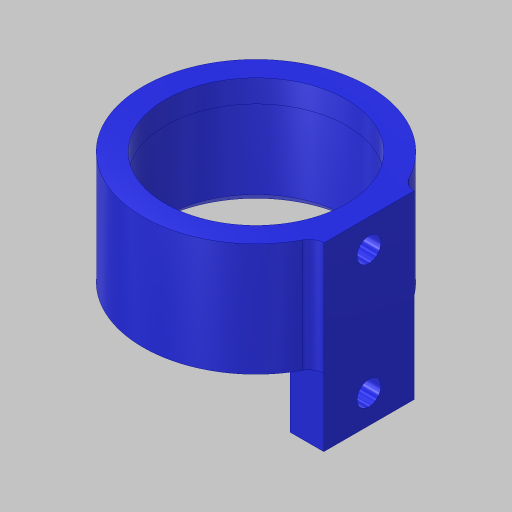
# Autodesk Inventor part: WL-008
Saved by Autodesk Inventor 2023.5 (Build 275446000, 446)
## iProperties
Created: 2025-02-22
Part Number: WL-008
Material: Aluminum 6061
Document SubType Name: Modeling
Designer: slick
Density: 2.7 g/cm^3
Appearance: Blue - Wall Paint - Glossy
Author: slick
Autodesk Inventor part; units mm, degrees
ref_plane "XZ Plane" through (0, 0, 0) normal (0, 1, 0) x (-1, 0, 0)
ref_plane "XY Plane" through (0, 0, 0) normal (0, 0, 1) x (1, 0, 0)
sketch "Sketch1" plane through (0, 0, 0) normal (0, 1, 0) x (-1, 0, 0)
  circle A0 centre (0, 0) radius 25.4
  circle A1 centre (0, 0) radius 31.75
  dimension "d0" = 50.8
  dimension "d1" = 63.5
  constraints: 2 centre point, 2 coincident
  measures "d0" diameter of A0
  measures "d1" diameter of A1
extrude "Extrusion1" add sketch "Sketch1" along normal blind 6.35
sketch "Sketch2" plane through (0, 0, 0) normal (0, -1, 0) x (1, 0, 0)
  circle A0 centre (0, 0) radius 25.654
  circle A1 centre (0, 0) radius 31.75 projected
  dimension "d4" = 51.308
  constraints: 1 centre point, 1 coincident
  measures "d4" diameter of A0
extrude "Extrusion2" add sketch "Sketch2" along normal blind 25.4
chamfer "Chamfer1" distance 3.175 angle 45 1 edges at (-25.654, -25.4, 0)
ref_plane "Work Plane1" through (31.75, 0, 0) normal (1, 0, 0) x (0, 1, 0)
sketch "Sketch5" plane through (31.75, 0, 0) normal (1, 0, 0) x (0, 1, 0)
  line L0 (-3.175, 31.75) -> (-34.925, 31.75) construction
  line L1 (-34.925, -31.75) -> (-3.175, -31.75) construction
  line L2 (-3.175, 31.75) -> (-34.925, -31.75) construction
  line L3 (-34.925, 31.75) -> (-3.175, -31.75) construction
  line L4 (0, 25.654) -> (0, -25.654) construction
  circle A0 centre (-19.05, 25.4) radius 3.35 construction
  circle A1 centre (-19.05, -25.4) radius 3.35 construction
  line L5 (-19.05, 25.4) -> (-19.05, -25.4) construction
  line L6 (-3.175, 31.75) -> (-3.175, -31.75) construction
  line L7 (-34.925, 31.75) -> (-34.925, -31.75) construction
  line L8 (-44.45, -12.7) -> (6.35, -12.7)
  line L9 (6.35, -12.7) -> (6.35, 12.7)
  line L10 (6.35, 12.7) -> (-44.45, 12.7)
  line L11 (-44.45, 12.7) -> (-44.45, -12.7)
  line L12 (-44.45, -12.7) -> (6.35, 12.7) construction
  line L13 (6.35, -12.7) -> (-44.45, 12.7) construction
  circle A2 centre (-1.5875, 0) radius 3.35
  circle A3 centre (-36.5125, 0) radius 3.35
  line L14 (-25.4, 31.75) -> (-25.4, -31.75) construction
  line L15 (6.35, -31.75) -> (6.35, 31.75) construction
  line L16 (6.35, -31.75) -> (6.35, 31.75) construction
  line L17 (6.35, 31.75) -> (-25.4, 31.75) construction
  line L18 (-25.4, 31.75) -> (6.35, 31.75) construction
  line L19 (-1.5875, 0) -> (-36.5125, 0) construction
  point P0 (0, 0)
  point P1 (6.35, 0)
  point P2 (-19.05, 0)
  point P3 (6.35, 0)
  point P4 (6.35, 0)
  point P5 (-9.525, 31.75)
  point P6 (-19.05, 0)
  point P7 (-44.45, 0)
  dimension "d27" = 63.5
  dimension "d28" = 50.8
  dimension "d29" = 6.7
  dimension "d35" = 25.4
  dimension "d36" = 34.925
  dimension "d37" = 50.8
  constraints: 30 end point, 10 midpoint, 4 centre point, 4 equal length, 4 horizontal alignment, 3 equal radius, 3 horizontal, 3 perpendicular, 1 coincident, 1 collinear, 1 vertical
  measures "d27" distance of L0.end L1.start
  measures "d28" distance of L5.start L5.end
  measures "d29" diameter of A0
  measures "d35" distance of L8.end L9.end
  measures "d36" distance of L19.start L19.end
  measures "d37" distance of point (-44.45, 0) point (6.35, 0)
extrude "Extrusion4" add sketch "Sketch5" against normal up to surface round surface about axis through (0, 0, 0) along (0, -1, 0) radius 25.654 far side no
extrude "Extrusion5" cut sketch "Sketch5" against normal blind 25.4 contours A2 | A3
fillet "Fillet1" radius 4.318 2 edges at (29.0994, -9.525, -12.7) (29.0994, -9.525, 12.7)
body "Solid1"
